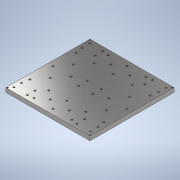
# Autodesk Inventor part: Mesa
Saved by Autodesk Inventor 2020 (Build 240168000, 168)
## iProperties
Created: 2020-05-08
Part Number: Mesa
Material: Steel, Mild
Document SubType Name: Modeling
Designer: Pipi
Density: 7.85 g/cm^3
Appearance: Semi-Polished
Mass: 3081.59 g
Surface Area: 994.228 cm^2
Volume: 392.56 cm^3
Author: Pipi
Autodesk Inventor part; units mm, degrees
ref_plane "YZ Plane" through (0, 0, 0) normal (1, 0, 0) x (0, 1, 0)
ref_plane "XZ Plane" through (0, 0, 0) normal (0, 1, 0) x (-1, 0, 0)
ref_plane "XY Plane" through (0, 0, 0) normal (0, 0, 1) x (1, 0, 0)
sketch "Boceto1" plane through (0, 0, 0) normal (0, 1, 0) x (-1, 0, 0)
  line L0 (-0.5, 0) -> (199.5, 0)
  line L1 (199.5, 0) -> (199.5, -200)
  line L2 (199.5, -200) -> (-0.5, -200)
  line L3 (-0.5, 0) -> (-0.5, -200)
  line L4 (175, -50) -> (175, -150)
  line L5 (175, -150) -> (25, -150)
  line L6 (25, -150) -> (25, -50)
  line L7 (50, -175) -> (50, -25)
  line L8 (150, -175) -> (50, -175)
  line L9 (150, -25) -> (150, -175)
  line L10 (50, -25) -> (150, -25)
  line L11 (154.5, -5) -> (194.5, -5)
  line L12 (154.5, -5) -> (154.5, -33)
  line L13 (154.5, -33) -> (194.5, -33)
  line L14 (194.5, -33) -> (194.5, -5)
  line L15 (99.5, -100) -> (99.5, -105)
  line L16 (99.5, -105) -> (99.5, -95)
  line L17 (99.5, -95) -> (99.5, -100)
  line L18 (99.5, -100) -> (94.5, -100)
  line L19 (94.5, -100) -> (104.5, -100)
  line L20 (99.5, -100) -> (79.5, -100)
  line L21 (79.5, -100) -> (120.5, -100)
  line L22 (120.5, -100) -> (120.5, -120)
  line L23 (120.5, -120) -> (120.5, -80)
  line L24 (120.5, -80) -> (78.5, -80)
  line L25 (78.5, -80) -> (78.5, -120)
  line L26 (78.5, -120) -> (120.5, -120)
  line L27 (78.5, -80) -> (82.5, -80)
  line L28 (82.5, -80) -> (82.5, -120)
  line L29 (120.5, -120) -> (116.5, -120)
  line L30 (116.5, -120) -> (116.5, -80)
  line L31 (82.5, -80) -> (82.5, -90)
  line L32 (82.5, -90) -> (116.5, -90)
  line L33 (82.5, -120) -> (82.5, -110)
  line L34 (82.5, -110) -> (116.5, -110)
  circle A0 centre (82.5, -90) radius 2
  circle A1 centre (82.5, -110) radius 2
  circle A2 centre (116.5, -110) radius 2
  circle A3 centre (116.5, -90) radius 2
  line L35 (194.5, -5) -> (190.5, -5)
  line L36 (190.5, -5) -> (190.5, -33)
  line L37 (154.5, -5) -> (158.5, -5)
  line L38 (158.5, -5) -> (158.5, -33)
  line L39 (158.5, -5) -> (158.5, -10)
  line L40 (158.5, -33) -> (158.5, -28)
  line L41 (158.5, -28) -> (190.5, -28)
  line L42 (158.5, -10) -> (190.5, -10)
  circle A4 centre (190.5, -10) radius 2
  circle A5 centre (158.5, -10) radius 2
  circle A6 centre (158.5, -28) radius 2
  circle A7 centre (190.5, -28) radius 2
  line L43 (44.5, -5) -> (4.5, -5)
  line L44 (44.5, -5) -> (44.5, -33)
  line L45 (44.5, -33) -> (4.5, -33)
  line L46 (4.5, -33) -> (4.5, -5)
  line L47 (4.5, -5) -> (8.5, -5)
  line L48 (8.5, -5) -> (8.5, -33)
  line L49 (44.5, -5) -> (40.5, -5)
  line L50 (40.5, -5) -> (40.5, -33)
  line L51 (40.5, -5) -> (40.5, -10)
  line L52 (40.5, -33) -> (40.5, -28)
  line L53 (40.5, -28) -> (8.5, -28)
  line L54 (40.5, -10) -> (8.5, -10)
  circle A8 centre (8.5, -10) radius 2
  circle A9 centre (40.5, -10) radius 2
  circle A10 centre (40.5, -28) radius 2
  circle A11 centre (8.5, -28) radius 2
  line L55 (155, -195) -> (194.5, -195)
  line L56 (155, -195) -> (155, -167)
  line L57 (155, -167) -> (194.5, -167)
  line L58 (194.5, -167) -> (194.5, -195)
  line L59 (194.5, -195) -> (190.5, -195)
  line L60 (190.5, -195) -> (190.5, -167)
  line L61 (155, -195) -> (159, -195)
  line L62 (159, -195) -> (159, -167)
  line L63 (159, -195) -> (159, -190)
  line L64 (159, -167) -> (159, -172)
  line L65 (159, -172) -> (190.5, -172)
  line L66 (159, -190) -> (190.5, -190)
  circle A12 centre (190.5, -190) radius 2
  circle A13 centre (159, -190) radius 2
  circle A14 centre (159, -172) radius 2
  circle A15 centre (190.5, -172) radius 2
  line L67 (44.5, -195) -> (4.5, -195)
  line L68 (44.5, -195) -> (44.5, -167)
  circle A16 centre (40.5, -172) radius 2
  line L69 (44.5, -167) -> (4.5, -167)
  line L70 (4.5, -167) -> (4.5, -195)
  line L71 (40.5, -167) -> (40.5, -172)
  circle A17 centre (40.5, -190) radius 2
  line L72 (40.5, -195) -> (40.5, -167)
  line L73 (40.5, -195) -> (40.5, -190)
  line L74 (40.5, -172) -> (8.5, -172)
  circle A18 centre (8.5, -172) radius 2
  line L75 (40.5, -190) -> (8.5, -190)
  line L76 (8.5, -195) -> (8.5, -167)
  circle A19 centre (8.5, -190) radius 2
  line L77 (4.5, -195) -> (8.5, -195)
  line L78 (44.5, -195) -> (40.5, -195)
  circle A20 centre (187.5, -45) radius 2
  circle A21 centre (187.5, -100) radius 2
  circle A22 centre (187.5, -155) radius 2
  circle A23 centre (144.5, -188) radius 2
  circle A24 centre (99.5, -188) radius 2
  circle A25 centre (54.5, -188) radius 2
  circle A26 centre (11.5, -45) radius 2
  circle A27 centre (11.5, -100) radius 2
  circle A28 centre (11.5, -155) radius 2
  circle A29 centre (144.5, -12) radius 2
  circle A30 centre (99.5, -12) radius 2
  circle A31 centre (54.5, -12) radius 2
  circle A32 centre (144.5, -155) radius 2
  circle A33 centre (142.5, -45) radius 2
  circle A34 centre (54.5, -45) radius 2
  circle A35 centre (54.5, -100) radius 2
  circle A36 centre (144.5, -100) radius 2
  circle A37 centre (54.5, -155) radius 2
  circle A38 centre (99.5, -155) radius 2
  circle A39 centre (100, -45) radius 2
  circle A40 centre (197.5, -198) radius 1.5
  circle A41 centre (197.5, -2) radius 1.5
  circle A42 centre (1.5, -2) radius 1.5
  circle A43 centre (1.5, -198) radius 1.5
  line L79 (187.5, -45) -> (11.5, -45)
  circle A44 centre (122, -172) radius 2
  circle A45 centre (166.5, -127.5) radius 2
  circle A46 centre (166.5, -72.5) radius 2
  circle A47 centre (77, -172) radius 2
  circle A48 centre (32.5, -127.5) radius 2
  circle A49 centre (32.5, -72.5) radius 2
  circle A50 centre (122, -28) radius 2
  circle A51 centre (77, -28) radius 2
  point P0 (0, 0)
  dimension "d0" = 200
  dimension "d1" = 200
  dimension "d2" = 200
  dimension "d6" = 100
  dimension "d7" = 150
  dimension "d8" = 100
  dimension "d30" = 28
  dimension "d98" = 4
  dimension "d99" = 4
  dimension "d100" = 10
  dimension "d101" = 10
  dimension "d102" = 4
  dimension "d103" = 4
  dimension "d104" = 4
  dimension "d105" = 4
  dimension "d116" = 4
  dimension "d117" = 4
  dimension "d118" = 5
  dimension "d119" = 5
  dimension "d120" = 4
  dimension "d121" = 4
  dimension "d122" = 4
  dimension "d123" = 4
  dimension "d124" = 5
  dimension "d166" = 20
  dimension "d167" = 20
  dimension "d236" = 21
  dimension "d237" = 100
  dimension "d238" = 21
  dimension "d264" = 4
  dimension "d265" = 4
  dimension "d266" = 4
  dimension "d267" = 4
  dimension "d268" = 4
  dimension "d269" = 4
  dimension "d270" = 12
  dimension "d271" = 12
  dimension "d272" = 12
  dimension "d273" = 100
  dimension "d274" = 55
  dimension "d275" = 55
  dimension "d276" = 12
  dimension "d277" = 12
  dimension "d278" = 100
  dimension "d279" = 45
  dimension "d280" = 45
  dimension "d284" = 4
  dimension "d285" = 4
  dimension "d286" = 4
  dimension "d287" = 4
  dimension "d288" = 4
  dimension "d289" = 4
  dimension "d290" = 4
  dimension "d291" = 4
  dimension "d312" = 3
  dimension "d313" = 2
  dimension "d314" = 2
  dimension "d315" = 3
  dimension "d316" = 3
  dimension "d317" = 3
  dimension "d318" = 2
  dimension "d319" = 2
  dimension "d320" = 2
  dimension "d321" = 2
  constraints: 160 end point, 52 centre point, 44 point on line, 20 coincident, 19 perpendicular, 12 symmetric about line, 3 horizontal, 2 vertical, 1 collinear, 12 other
  measures "d0" distance of L0.start L0.end
  measures "d1" distance of L0.end L1.end
  measures "d2" distance of L1.end L2.end
  measures "d6" distance of L4.start L4.end
  measures "d7" distance of L4.end L6.start
  measures "d8" distance of L10.start L10.end
  measures "d30" distance of L11.start L12.end
  measures "d98" distance of L24.end L27.end
  measures "d99" distance of L22.end L29.end
  measures "d100" distance of L27.end L31.end
  measures "d101" distance of L28.end L33.end
  measures "d102" diameter of A0
  measures "d103" diameter of A1
  measures "d104" diameter of A2
  measures "d105" diameter of A3
  measures "d116" distance of L11.end L35.end
  measures "d117" distance of L11.start L37.end
  measures "d118" distance of L37.end L39.end
  measures "d119" distance of L38.end L40.end
  measures "d120" diameter of A4
  measures "d121" diameter of A5
  measures "d122" diameter of A6
  measures "d123" diameter of A7
  measures "d124" distance between parallel lines of L0 L11
  measures "d166" distance from line of L24 L15.start
  measures "d167" distance between parallel lines of L26 L19
  measures "d236" distance from line of L25 L15.start
  measures "d237" distance from line of L3 L15.start
  measures "d238" distance between parallel lines of L15 L23
  measures "d264" diameter of A20
  measures "d265" diameter of A21
  measures "d266" diameter of A22
  measures "d267" diameter of A23
  measures "d268" diameter of A24
  measures "d269" diameter of A25
  measures "d270" distance from line of L1 A22.centre
  measures "d271" distance from line of L1 A21.centre
  measures "d272" distance from line of L1 L79.start
  measures "d273" distance from line of L0 A21.centre
  measures "d274" distance of L79.start A21.centre
  measures "d275" distance of A22.centre A21.centre
  measures "d276" distance from line of L2 A23.centre
  measures "d277" distance from line of L2 A25.centre
  measures "d278" distance from line of L3 A24.centre
  measures "d279" distance of A24.centre A23.centre
  measures "d280" distance of A25.centre A24.centre
  measures "d284" diameter of A32
  measures "d285" diameter of A33
  measures "d286" diameter of A34
  measures "d287" diameter of A35
  measures "d288" diameter of A36
  measures "d289" diameter of A37
  measures "d290" diameter of A38
  measures "d291" diameter of A39
  measures "d312" diameter of A40
  measures "d313" distance from line of L1 A40.centre
  measures "d314" distance from line of L2 A40.centre
  measures "d315" diameter of A41
  measures "d316" diameter of A42
  measures "d317" diameter of A43
  measures "d318" distance from line of L2 A43.centre
  measures "d319" distance from line of L3 A43.centre
  measures "d320" distance from line of L3 A42.centre
  measures "d321" distance from line of L0 A42.centre
extrude "Extrusión1" add sketch "Boceto1" along normal blind 10 contours L0 L1 L2 L3 | L9 L8 L7 L5 | L5 L7 L79 A34 A39 A33 L9 | L79 A33 A39 A34 L7 L10 L9 | L11 L38 A5 A6 L13 L12 | L11 L36 A4 L42 A5 L38 | L11 L14 L13 L36 A7 A4 | L38 A6 L41 A7 L36 L13 | L42 A4 L36 A7 L41 A6 L38 A5 | L19 L21 L30 A2 L34 A1 L28 L20 L18 | L18 L20 L28 A0 L32 A3 L30 L21 L19 | L28 A1 L26 L25 L24 A0 | L30 A3 L24 L23 L21 | L21 L22 L26 L30 A2 | L28 L24 L30 A3 L32 A0 | L34 A2 L30 L26 L28 A1 | L44 L45 L50 A10 A9 L43 | L50 A9 L54 A8 L48 L43 | L48 A8 A11 L45 L46 L43 | L45 L48 A11 L53 A10 L50 | A9 L50 A10 L53 A11 L48 A8 L54 | L56 L57 L62 A14 A13 L55 | L62 A13 L66 A12 L60 L55 | L60 A12 A15 L57 L58 L55 | L57 L60 A15 L65 A14 L62 | L62 A14 L65 A15 L60 A12 L66 A13 | L67 L72 A17 A16 L71 L69 L68 | L67 L76 A19 L75 A17 L72 | L67 L70 L69 L76 A18 A19 | L71 A16 L74 A18 L76 L69 | L75 A19 L76 A18 L74 A16 L72 A17
thread "Rosca46" size "M4x0.7" class "6H" standard "ISO Metric profile" length 10
thread "Rosca47" size "M3x0.5" class "6H" standard "ISO Metric profile" length 10
thread "Rosca48" size "M4x0.7" class "6H" standard "ISO Metric profile" length 10
thread "Rosca49" size "M4x0.7" class "6H" standard "ISO Metric profile" length 10
thread "Rosca50" size "M4x0.7" class "6H" standard "ISO Metric profile" length 10
thread "Rosca51" size "M4x0.7" class "6H" standard "ISO Metric profile" length 10
thread "Rosca52" size "M4x0.7" class "6H" standard "ISO Metric profile" length 10
thread "Rosca53" size "M4x0.7" class "6H" standard "ISO Metric profile" length 10
thread "Rosca54" size "M4x0.7" class "6H" standard "ISO Metric profile" length 10
thread "Rosca55" size "M4x0.7" class "6H" standard "ISO Metric profile" length 10
thread "Rosca56" size "M4x0.7" class "6H" standard "ISO Metric profile" length 10
thread "Rosca57" size "M4x0.7" class "6H" standard "ISO Metric profile" length 10
thread "Rosca58" size "M4x0.7" class "6H" standard "ISO Metric profile" length 10
thread "Rosca59" size "M4x0.7" class "6H" standard "ISO Metric profile" length 10
thread "Rosca60" size "M4x0.7" class "6H" standard "ISO Metric profile" length 10
thread "Rosca61" size "M3x0.5" class "6H" standard "ISO Metric profile" length 10
thread "Rosca62" size "M4x0.7" class "6H" standard "ISO Metric profile" length 10
thread "Rosca63" size "M4x0.7" class "6H" standard "ISO Metric profile" length 10
thread "Rosca64" size "M4x0.7" class "6H" standard "ISO Metric profile" length 10
thread "Rosca65" size "M4x0.7" class "6H" standard "ISO Metric profile" length 10
thread "Rosca66" size "M4x0.7" class "6H" standard "ISO Metric profile" length 10
thread "Rosca67" size "M4x0.7" class "6H" standard "ISO Metric profile" length 10
thread "Rosca68" size "M4x0.7" class "6H" standard "ISO Metric profile" length 10
thread "Rosca69" size "M4x0.7" class "6H" standard "ISO Metric profile" length 10
thread "Rosca70" size "M4x0.7" class "6H" standard "ISO Metric profile" length 10
thread "Rosca71" size "M3x0.5" class "6H" standard "ISO Metric profile" length 10
thread "Rosca72" size "M4x0.7" class "6H" standard "ISO Metric profile" length 10
thread "Rosca73" size "M4x0.7" class "6H" standard "ISO Metric profile" length 10
thread "Rosca74" size "M4x0.7" class "6H" standard "ISO Metric profile" length 10
thread "Rosca75" size "M4x0.7" class "6H" standard "ISO Metric profile" length 10
thread "Rosca76" size "M4x0.7" class "6H" standard "ISO Metric profile" length 10
thread "Rosca77" size "M4x0.7" class "6H" standard "ISO Metric profile" length 10
thread "Rosca78" size "M4x0.7" class "6H" standard "ISO Metric profile" length 10
thread "Rosca79" size "M4x0.7" class "6H" standard "ISO Metric profile" length 10
thread "Rosca80" size "M4x0.7" class "6H" standard "ISO Metric profile" length 10
thread "Rosca81" size "M4x0.7" class "6H" standard "ISO Metric profile" length 10
thread "Rosca82" size "M4x0.7" class "6H" standard "ISO Metric profile" length 10
thread "Rosca83" size "M3x0.5" class "6H" standard "ISO Metric profile" length 10
thread "Rosca84" size "M4x0.7" class "6H" standard "ISO Metric profile" length 10
thread "Rosca85" size "M4x0.7" class "6H" standard "ISO Metric profile" length 10
thread "Rosca86" size "M4x0.7" class "6H" standard "ISO Metric profile" length 10
thread "Rosca87" size "M4x0.7" class "6H" standard "ISO Metric profile" length 10
thread "Rosca88" size "M4x0.7" class "6H" standard "ISO Metric profile" length 10
thread "Rosca89" size "M4x0.7" class "6H" standard "ISO Metric profile" length 10
sketch "Boceto3" plane through (0, 10, 0) normal (0, 1, 0) x (1, 0, 0)
  circle A0 centre (-54.5, 12) radius 2 projected
  point P0 (0, 0)
thread "Thread90" size "M4x0.7" class "6H" standard "ISO Metric profile" length 25
thread "Thread91" size "M4x0.7" class "6H" standard "ISO Metric profile" length 25
thread "Thread92" size "M4x0.7" class "6H" standard "ANSI Metric M Profile" length 25
thread "Thread93" size "M4x0.7" class "6H" standard "ISO Metric profile" length 25
thread "Thread94" size "M4x0.7" class "6H" standard "ISO Metric profile" length 25
thread "Thread95" size "M4x0.7" class "6H" standard "ISO Metric profile" length 25
thread "Thread96" size "M4x0.7" class "6H" standard "ISO Metric profile" length 25
thread "Thread97" size "M4x0.7" class "6H" standard "ISO Metric profile" length 25
